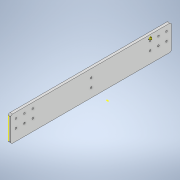
# Autodesk Inventor part: Holder e Holder gripper
Saved by Autodesk Inventor 2021 (Build 250183000, 183)
## iProperties
Created: 2025-09-23
Part Number: Holder e Holder gripper
Material: Generic
Document SubType Name: Modeling
Designer: Naufal K
Density: 1 g/cm^3
Appearance: Default
Author: Naufal K
Autodesk Inventor part; units mm, degrees
ref_plane "YZ Plane" through (0, 0, 0) normal (1, 0, 0) x (0, 1, 0)
ref_plane "XZ Plane" through (0, 0, 0) normal (0, 1, 0) x (-1, 0, 0)
ref_plane "XY Plane" through (0, 0, 0) normal (0, 0, 1) x (1, 0, 0)
sketch "Sketch2" plane through (0, 0, 0) normal (1, 0, 0) x (0, 1, 0)
  line L0 (45.0919, 116.9004) -> (15.0919, 116.9004)
  line L1 (15.0919, 116.9004) -> (15.0919, -73.0996)
  line L2 (15.0919, -73.0996) -> (45.0919, -73.0996)
  line L3 (45.0919, -73.0996) -> (45.0919, 116.9004)
  point P0 (0, 0)
  dimension "d0" = 30
  dimension "d1" = 190
  constraints: 8 end point, 2 parallel, 1 horizontal, 1 perpendicular
  measures "d0" distance of L2.end L1.end
  measures "d1" distance of L1.end L0.end
extrude "Extrusion1" add sketch "Sketch2" along normal blind 3
sketch "Sketch4" plane through (0, 0, 0) normal (-1, 0, 0) x (0, 0, 1)
  circle A0 centre (-67.0996, 38.6968) radius 2
  line L0 (-73.0996, 15.0919) -> (-73.0996, 45.0919) projected
  point P0 (0, 0)
  dimension "d7" = 4
  dimension "d8" = 6
  constraints: 1 centre point
  measures "d7" diameter of A0
  measures "d8" distance from line of L0 A0.centre
extrude "Extrusion3" cut sketch "Sketch4" against normal blind 1
sketch "Sketch5" plane through (1, 38.6968, -67.0996) normal (-1, 0, 0) x (0, 0, 1)
  circle A0 centre (0, 0) radius 1
  point P0 (67.0996, -38.6968)
  dimension "d11" = 2
  constraints: 1 centre point
  measures "d11" diameter of A0
extrude "Extrusion4" cut sketch "Sketch5" against normal blind 2
sketch "Sketch6" plane through (0, 0, 0) normal (-1, 0, 0) x (0, 0, 1)
  circle A0 centre (-67.0996, 28.6968) radius 1
  circle A1 centre (-67.0996, 28.6968) radius 2
  circle A2 centre (-67.0996, 38.6968) radius 2 projected
  point P0 (0, 0)
  dimension "d14" = 2
  dimension "d15" = 4
  dimension "d17" = 10
  constraints: 2 centre point, 1 coincident
  measures "d14" diameter of A0
  measures "d15" diameter of A1
  measures "d17" distance of A0.centre A2.centre
extrude "Extrusion5" cut sketch "Sketch6" against normal blind 1 contours A0 | A1
sketch "Sketch7" plane through (1, 28.6968, -67.0996) normal (-1, 0, 0) x (0, 0, 1)
  circle A0 centre (0, 0) radius 1
  point P0 (67.0996, -28.6968)
  dimension "d20" = 2
  constraints: 1 centre point
  measures "d20" diameter of A0
extrude "Extrusion6" cut sketch "Sketch7" against normal blind 2
sketch "Sketch8" plane through (0, 106.1298, -18.9436) normal (-1, 0, 0) x (0, 1, 0)
  circle A0 centre (-67.4331, 38.6843) radius 2
  line L0 (-73.0996, 15.0919) -> (-73.5243, 45.0873)
  circle A1 centre (-67.4331, 48.156) radius 2 projected
  point P0 (0, 0)
  dimension "d23" = 4
  dimension "d24" = 6
  dimension "d45" = 9.4717
  dimension "d46" = 9.4717
  constraints: 2 end point, 1 centre point
  measures "d23" diameter of A0
  measures "d24" distance from line of L0 A0.centre
  measures "d45" distance of A0.centre A1.centre
  measures "d46" distance of A0.centre A1.centre
extrude "Extrusion7" cut sketch "Sketch8" against normal blind 1 contours A0
sketch "Sketch9" plane through (1, 38.6968, -57.6279) normal (-1, 0, 0) x (0, 0, 1)
  circle A0 centre (0, 0) radius 1
  point P0 (67.0996, -38.6968)
  dimension "d28" = 2
  constraints: 1 centre point
  measures "d28" diameter of A0
extrude "Extrusion8" cut sketch "Sketch9" against normal blind 2
sketch "Sketch10" plane through (0, 30.0919, 21.9004) normal (-1, 0, 0) x (0, -1, 0)
  circle A0 centre (1.395, -79.4792) radius 1
  circle A1 centre (1.395, -79.4792) radius 2
  circle A2 centre (-8.6049, -79.5283) radius 2 projected
  circle A3 centre (1.3951, -89) radius 2 projected
  point P0 (0, 0)
  dimension "d33" = 2
  dimension "d32" = 4
  dimension "d34" = 10
  dimension "d47" = 9.5208
  dimension "d48" = 9.5208
  constraints: 2 centre point, 1 coincident
  measures "d33" diameter of A0
  measures "d32" diameter of A1
  measures "d34" distance of A0.centre A2.centre
  measures "d47" distance of A1.centre A3.centre
  measures "d48" distance of A0.centre A3.centre
extrude "Extrusion9" cut sketch "Sketch10" against normal blind 1 contours A0 | A1
sketch "Sketch12" plane through (1, 28.6969, -57.5789) normal (-1, 0, 0) x (0, 0, 1)
  circle A0 centre (0, 0) radius 1
  point P0 (57.5789, -28.6969)
  dimension "d42" = 2
  constraints: 1 centre point
  measures "d42" diameter of A0
extrude "Extrusion11" cut sketch "Sketch12" against normal blind 2
sketch "Sketch14" plane through (0, -38.3101, -86.469) normal (-1, 0, 0) x (0, -1, 0)
  circle A0 centre (-67.007, 38.6968) radius 2
  line L0 (-73.0996, 15.0919) -> (-72.982, 45.0906)
  circle A1 centre (-67.007, 28.8901) radius 2 projected
  point P0 (0, 0)
  dimension "d49" = 4
  dimension "d50" = 6
  dimension "d71" = 9.8066
  constraints: 2 end point, 1 centre point
  measures "d49" diameter of A0
  measures "d50" distance from line of L0 A0.centre
  measures "d71" distance of A1.centre A0.centre
extrude "Extrusion12" cut sketch "Sketch14" against normal blind 1 contours A0
sketch "Sketch15" plane through (1, 28.6969, -47.7722) normal (-1, 0, 0) x (0, 0, 1)
  circle A0 centre (0, 0) radius 1
  point P0 (67.0996, -38.6968)
  dimension "d54" = 2
  constraints: 1 centre point
  measures "d54" diameter of A0
extrude "Extrusion13" cut sketch "Sketch15" against normal blind 2
sketch "Sketch16" plane through (0, 30.0919, 21.9004) normal (-1, 0, 0) x (0, -1, 0)
  circle A0 centre (-8.605, -69.6678) radius 1
  circle A1 centre (-8.605, -69.6678) radius 2
  circle A2 centre (1.395, -69.6726) radius 2 projected
  circle A3 centre (-8.6049, -79.5283) radius 2 projected
  circle A4 centre (1.395, -79.4792) radius 2 projected
  point P0 (0, 0)
  dimension "d59" = 2
  dimension "d58" = 4
  dimension "d60" = 10
  dimension "d68" = 9.8605
  dimension "d69" = 9.8066
  constraints: 2 centre point, 1 coincident
  measures "d59" diameter of A0
  measures "d58" diameter of A1
  measures "d60" distance of A0.centre A2.centre
  measures "d68" distance of A1.centre A3.centre
  measures "d69" distance of A4.centre A2.centre
extrude "Extrusion14" cut sketch "Sketch16" against normal blind 1 contours A0 | A1
sketch "Sketch17" plane through (1, 38.6969, -47.7675) normal (-1, 0, 0) x (0, 0, 1)
  circle A0 centre (0, 0) radius 1
  point P0 (67.0996, -28.6968)
  dimension "d64" = 2
  constraints: 1 centre point
  measures "d64" diameter of A0
extrude "Extrusion15" cut sketch "Sketch17" against normal blind 2
fillet "Fillet1" radius 2 4 edges at (1.5, 45.0919, 116.9004) (1.5, 15.0919, 116.9004) (1.5, 45.0919, -73.0996) (1.5, 15.0919, -73.0996)
sketch "Sketch18" plane through (0, 0, 0) normal (-1, 0, 0) x (0, 0, 1)
  circle A0 centre (110.9004, 38.6968) radius 2
  line L0 (116.9004, 43.0919) -> (116.9004, 17.0919) projected
  point P0 (0, 0)
  dimension "d73" = 4
  dimension "d79" = 6
  constraints: 1 centre point
  measures "d73" diameter of A0
  measures "d79" distance from line of L0 A0.centre
extrude "Extrusion16" cut sketch "Sketch18" against normal blind 1
sketch "Sketch19" plane through (1, 38.6968, 110.9004) normal (-1, 0, 0) x (0, 0, 1)
  circle A0 centre (0, 0) radius 1
  point P0 (-110.9004, -38.6968)
  dimension "d76" = 2
  constraints: 1 centre point
  measures "d76" diameter of A0
extrude "Extrusion17" cut sketch "Sketch19" against normal blind 2
sketch "Sketch21" plane through (0, 0, 0) normal (-1, 0, 0) x (0, 0, 1)
  circle A0 centre (110.9004, 28.6968) radius 1
  circle A1 centre (110.9004, 38.6968) radius 1 projected
  point P0 (0, 0)
  dimension "d84" = 2
  dimension "d90" = 10
  constraints: 1 centre point
  measures "d84" diameter of A0
  measures "d90" distance of A1.centre A0.centre
extrude "Extrusion19" cut sketch "Sketch21" against normal blind 3 contours A0
sketch "Sketch22" plane through (0, 0, 0) normal (-1, 0, 0) x (0, 0, 1)
  circle A0 centre (110.9004, 28.6968) radius 1 projected
  circle A1 centre (110.9004, 28.6968) radius 2
  point P0 (0, 0)
  dimension "d87" = 4
  constraints: 1 centre point, 1 coincident
  measures "d87" diameter of A1
extrude "Extrusion20" cut sketch "Sketch22" against normal blind 1
sketch "Sketch23" plane through (0, 0, 0) normal (-1, 0, 0) x (0, 0, 1)
  circle A0 centre (100.9004, 38.6968) radius 2
  circle A1 centre (110.9004, 38.6968) radius 1 projected
  point P0 (0, 0)
  dimension "d93" = 10
  constraints: 1 centre point
  measures "d93" distance of A1.centre A0.centre
extrude "Extrusion21" cut sketch "Sketch23" against normal blind 1 contours A0
sketch "Sketch24" plane through (0, 0, 0) normal (-1, 0, 0) x (0, 0, 1)
  circle A0 centre (100.9004, 28.6968) radius 2
  circle A1 centre (110.9004, 28.6968) radius 2 projected
  point P0 (0, 0)
  dimension "d97" = 10
  constraints: 1 centre point
  measures "d97" distance of A1.centre A0.centre
extrude "Extrusion22" cut sketch "Sketch24" against normal blind 1 contours A0
sketch "Sketch25" plane through (0, 0, 0) normal (-1, 0, 0) x (0, 0, 1)
  circle A0 centre (90.9004, 38.6968) radius 2
  circle A1 centre (100.9004, 38.6968) radius 2 projected
  point P0 (0, 0)
  dimension "d98" = 10
  constraints: 1 centre point
  measures "d98" distance of A1.centre A0.centre
sketch "Sketch26" plane through (1, 28.6968, 100.9004) normal (-1, 0, 0) x (0, 0, 1)
  point P0 (-100.9004, -28.6968)
sketch "Sketch27" plane through (0, 0, 0) normal (-1, 0, 0) x (0, 0, 1)
  circle A0 centre (90.9004, 28.6968) radius 2
  circle A1 centre (100.9004, 28.6968) radius 2 projected
  point P0 (0, 0)
  dimension "d99" = 10
  constraints: 1 centre point
  measures "d99" distance of A1.centre A0.centre
extrude "Extrusion23" cut sketch "Sketch25" against normal blind 1 contours A0
extrude "Extrusion24" cut sketch "Sketch27" against normal blind 1 contours A0
sketch "Sketch28" plane through (0, 0, 0) normal (-1, 0, 0) x (0, 0, 1)
  point P0 (0, 0)
sketch "Sketch29" plane through (1, 38.6968, 90.9004) normal (-1, 0, 0) x (0, 0, 1)
  circle A0 centre (0, 0) radius 1
  circle A1 centre (0, -10) radius 2 projected
  circle A2 centre (0, -10) radius 1
  circle A3 centre (10, -10) radius 2 projected
  circle A4 centre (10, -10) radius 1
  circle A5 centre (10, 0) radius 2 projected
  circle A6 centre (10, 0) radius 1
  point P0 (-90.9004, -38.6968)
  dimension "d104" = 2
  dimension "d105" = 2
  constraints: 4 centre point, 3 coincident
  measures "d104" diameter of A0
  measures "d105" diameter of A2
extrude "Extrusion25" cut sketch "Sketch29" against normal blind 2 contours A0 | A2 | A4 | A6
sketch "Sketch30" plane through (0, 0, 0) normal (-1, 0, 0) x (0, 0, 1)
  point P0 (0, 0)
sketch "Sketch31" plane through (0, 0, 0) normal (-1, 0, 0) x (0, 0, 1)
  line L0 (21.9004, 37.6669) -> (23.6324, 36.6669)
  line L1 (23.6324, 36.6669) -> (23.6324, 34.6669)
  line L2 (23.6324, 34.6669) -> (21.9004, 33.6669)
  line L3 (21.9004, 33.6669) -> (20.1683, 34.6669)
  line L4 (20.1683, 34.6669) -> (20.1683, 36.6669)
  line L5 (20.1683, 36.6669) -> (21.9004, 37.6669)
  line L6 (21.9004, 27.6669) -> (23.6324, 26.6669)
  line L7 (23.6324, 26.6669) -> (23.6324, 24.6669)
  line L8 (23.6324, 24.6669) -> (21.9004, 23.6669)
  line L9 (21.9004, 23.6669) -> (20.1683, 24.6669)
  line L10 (20.1683, 24.6669) -> (20.1683, 26.6669)
  line L11 (20.1683, 26.6669) -> (21.9004, 27.6669)
  point P0 (0, 0)
  point P1 (21.9004, 35.6669)
  point P2 (21.9004, 25.6669)
  dimension "d108" = 4
  dimension "d109" = 4
  dimension "d110" = 6
  constraints: 24 end point, 26 other
  measures "d108" distance of L2.end L0.start
  measures "d109" distance of L8.end L6.start
  measures "d110" distance of L6.start L2.end
extrude "Extrusion26" cut sketch "Sketch31" against normal blind 1
sketch "Sketch32" plane through (1, 0, 0) normal (-1, 0, 0) x (0, 0, 1)
  circle A0 centre (21.9004, 25.6669) radius 1
  circle A1 centre (21.9004, 35.6669) radius 1
  point P0 (0, 0)
  constraints: 2 centre point
extrude "Extrusion27" cut sketch "Sketch32" against normal blind 2
sketch "Sketch33" plane through (0, 0, 0) normal (-1, 0, 0) x (0, 0, 1)
  circle A0 centre (-67.0996, 38.6968) radius 1 projected
  line L0 (116.9004, 43.0919) -> (116.9004, 17.0919) projected
  point P0 (0, 0)
body "Solid1"
